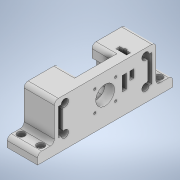
# Autodesk Inventor part: Y_motor_mount
Saved by Autodesk Inventor 2020 (Build 240168000, 168)
## iProperties
Created: 2022-04-26
Part Number: Y_motor_mount
Material: Ogólny
Document SubType Name: Modeling
Designer: mikoma
Density: 1 g/cm^3
Appearance: Domyślna
Author: mikoma
Autodesk Inventor part; units mm, degrees
ref_plane "YZ Plane" through (0, 0, 0) normal (1, 0, 0) x (0, 1, 0)
ref_plane "XZ Plane" through (0, 0, 0) normal (0, 1, 0) x (-1, 0, 0)
ref_plane "XY Plane" through (0, 0, 0) normal (0, 0, 1) x (1, 0, 0)
sketch "Szkic1" plane through (0, 0, 0) normal (1, 0, 0) x (0, 1, 0)
  circle A0 centre (0, 0) radius 14
  arc A1 (15.7574, 63.5) -> (15.0197, 62.3339) centre (20, 60) ccw construction
  arc A2 (-20.25, 65.4943) -> (-15.0197, 62.3339) centre (-20, 60) ccw
  line L0 (20.25, 69.5) -> (-20.25, 69.5)
  line L1 (-20.25, 69.5) -> (-20.25, 65.4943)
  line L2 (-20.25, 63.5) -> (-15.7574, 63.5) construction
  line L3 (20.25, 63.5) -> (20.25, 65.4943) construction
  line L4 (15.7574, 63.5) -> (20.25, 63.5) construction
  line L5 (20.25, 65.4943) -> (20.25, 69.5)
  line L6 (-20.25, 65.4943) -> (-20.25, 63.5) construction
  line L7 (-15.7574, 63.5) -> (-13, 63.5) construction
  arc A3 (20.25, 65.4943) -> (15.7574, 63.5) centre (20, 60) ccw construction
  arc A4 (-15.7574, 63.5) -> (-20.25, 65.4943) centre (-20, 60) ccw construction
  line L8 (-15.0197, 62.3339) -> (-13, 63.5)
  line L9 (13, 63.5) -> (15.0197, 62.3339)
  arc A5 (15.0197, 62.3339) -> (20.25, 65.4943) centre (20, 60) ccw
  line L10 (13, 63.5) -> (15.7574, 63.5) construction
  arc A6 (-15.0197, 62.3339) -> (-15.7574, 63.5) centre (-20, 60) ccw construction
  line L11 (-13, 63.5) -> (13, 63.5)
  line L12 (14, 0) -> (-14, 0) construction
  arc A7 (15.0197, -62.3339) -> (15.7574, -63.5) centre (20, -60) ccw construction
  arc A8 (-15.0197, -62.3339) -> (-20.25, -65.4943) centre (-20, -60) ccw
  line L13 (20.25, -69.5) -> (-20.25, -69.5)
  line L14 (-20.25, -69.5) -> (-20.25, -65.4943)
  line L15 (-20.25, -63.5) -> (-15.7574, -63.5) construction
  line L16 (20.25, -63.5) -> (20.25, -65.4943) construction
  line L17 (15.7574, -63.5) -> (20.25, -63.5) construction
  line L18 (20.25, -65.4943) -> (20.25, -69.5)
  line L19 (-20.25, -65.4943) -> (-20.25, -63.5) construction
  line L20 (-15.7574, -63.5) -> (-13, -63.5) construction
  arc A9 (15.7574, -63.5) -> (20.25, -65.4943) centre (20, -60) ccw construction
  arc A10 (-20.25, -65.4943) -> (-15.7574, -63.5) centre (-20, -60) ccw construction
  line L21 (-15.0197, -62.3339) -> (-13, -63.5)
  line L22 (13, -63.5) -> (15.0197, -62.3339)
  arc A11 (20.25, -65.4943) -> (15.0197, -62.3339) centre (20, -60) ccw
  line L23 (13, -63.5) -> (15.7574, -63.5) construction
  arc A12 (-15.7574, -63.5) -> (-15.0197, -62.3339) centre (-20, -60) ccw construction
  line L24 (-13, -63.5) -> (13, -63.5)
  line L25 (24.5, 75.5) -> (-19, 75.5)
  line L26 (-40, 75.5) -> (-40, -75.5)
  line L27 (-19, -75.5) -> (24.5, -75.5)
  line L28 (30.5, -69.5) -> (30.5, -31.5)
  arc A13 (30.5, 69.5) -> (24.5, 75.5) centre (24.5, 69.5) ccw
  arc A14 (24.5, -75.5) -> (30.5, -69.5) centre (24.5, -69.5) ccw
  line L29 (-40, 75.5) -> (-25, 75.5) construction
  line L30 (-25, 81.5) -> (-25, 94.5)
  line L31 (-31, 100.5) -> (-40, 100.5)
  line L32 (-40, 100.5) -> (-40, 75.5)
  arc A15 (-25, 94.5) -> (-31, 100.5) centre (-31, 94.5) ccw
  arc A16 (-25, 81.5) -> (-19, 75.5) centre (-19, 81.5) ccw
  line L33 (-40, -75.5) -> (-25, -75.5) construction
  line L34 (-25, -81.5) -> (-25, -94.5)
  line L35 (-31, -100.5) -> (-40, -100.5)
  line L36 (-40, -100.5) -> (-40, -75.5)
  arc A17 (-31, -100.5) -> (-25, -94.5) centre (-31, -94.5) ccw
  arc A18 (-19, -75.5) -> (-25, -81.5) centre (-19, -81.5) ccw
  circle A19 centre (15.5, 15.5) radius 1.75
  circle A20 centre (15.5, -15.5) radius 1.75
  circle A21 centre (-15.5, 15.5) radius 1.75
  circle A22 centre (-15.5, -15.5) radius 1.75
  line L37 (15.5, -15.5) -> (-15.5, 15.5) construction
  line L38 (15.5, 15.5) -> (-15.5, -15.5) construction
  circle A23 centre (15.5, 15.5) radius 3.5
  circle A24 centre (15.5, -15.5) radius 3.5
  circle A25 centre (-15.5, -15.5) radius 3.5
  circle A26 centre (-15.5, 15.5) radius 3.5
  line L39 (24.5, -25.5) -> (-15.5, -25.5)
  line L40 (-21.5, -19.5) -> (-21.5, 19.5)
  line L41 (-15.5, 25.5) -> (24.5, 25.5)
  line L42 (30.5, 25.5) -> (30.5, -25.5) construction
  arc A27 (30.5, -31.5) -> (24.5, -25.5) centre (24.5, -31.5) ccw
  arc A28 (-21.5, -19.5) -> (-15.5, -25.5) centre (-15.5, -19.5) ccw
  arc A29 (-15.5, 25.5) -> (-21.5, 19.5) centre (-15.5, 19.5) ccw
  line L43 (30.5, 31.5) -> (30.5, 69.5)
  arc A30 (24.5, 25.5) -> (30.5, 31.5) centre (24.5, 31.5) ccw
  line L44 (30.5, -31.5) -> (30.5, 31.5)
  point P0 (-25, 100.5)
  point P1 (-25, -100.5)
  dimension "d0" = 28
  dimension "d1" = 11
  dimension "d2" = 40
  dimension "d3" = 20
  dimension "d4" = 60
  dimension "d6" = 6
  dimension "d8" = 3.5
  dimension "d9" = 150
  dimension "d10" = 150
  dimension "d11" = 26
  dimension "d12" = 13
  dimension "d13" = 6
  dimension "d14" = 6
  dimension "d15" = 10.5
  dimension "d16" = 20
  dimension "d17" = 6
  dimension "d18" = 15
  dimension "d19" = 25
  dimension "d20" = 6
  dimension "d21" = 15
  dimension "d22" = 25
  dimension "d23" = 6
  dimension "d24" = 3.5
  dimension "d25" = 31
  dimension "d26" = 31
  dimension "d27" = 7
  dimension "d34" = 10
  dimension "d35" = 10
  dimension "d36" = 6
  dimension "d37" = 6
  dimension "d38" = 6
  dimension "d50" = 0.25
  dimension "d51" = 0.25
  constraints: 90 end point, 46 point on circle, 31 centre point, 20 tangent, 17 parallel, 14 symmetric about line, 13 point on line, 12 equal radius, 6 horizontal, 6 perpendicular, 5 coincident, 4 horizontal alignment, 2 midpoint, 2 vertical alignment, 1 collinear, 1 vertical, 6 other
  measures "d0" diameter of A0
  measures "d1" diameter of A1
  measures "d2" distance of A2.centre A1.centre
  measures "d3" horizontal distance of point (0, 0) A1.centre
  measures "d4" vertical distance of A1.centre point (0, 0)
  measures "d6" distance of L3.start L0.start
  measures "d8" distance from line of L2 A1.centre
  measures "d9" angle of L8 L7
  measures "d10" angle of L7 L9
  measures "d11" distance of L7.end L9.start
  measures "d12" horizontal distance of L9.start point (0, 0)
  measures "d13" distance between parallel lines of L0 L25
  measures "d14" distance between parallel lines of L13 L27
  measures "d15" distance from line of A1.centre L28
  measures "d16" distance from line of A2.centre L26
  measures "d17" radius of A13
  measures "d18" distance of point (-25, 100.5) L31.end
  measures "d19" distance of L29.end point (-25, 100.5)
  measures "d20" radius of A15
  measures "d21" distance of point (-25, -100.5) L35.end
  measures "d22" distance of L33.end point (-25, -100.5)
  measures "d23" radius of A17
  measures "d24" diameter of A19
  measures "d25" distance of L37.start L38.start
  measures "d26" distance of L38.end L37.start
  measures "d27" diameter of A23
  measures "d34" distance from line of L39 A24.centre
  measures "d35" distance from line of A23.centre L41
  measures "d36" distance from line of L38.end L40
  measures "d37" radius of A27
  measures "d38" radius of A30
  measures "d50" distance from line of A1.centre L5
  measures "d51" distance from line of L1 A2.centre
extrude "Wyciągnięcie proste1" add sketch "Szkic1" along normal blind 45 contours A0 | L1 L0 L5 A5 L9 L11 L8 A2 | L21 L24 L22 A11 L18 L13 L14 A8 | A13 L43 A30 L41 A29 L40 A28 L39 A27 L28 A14 L27 A18 L34 A17 L35 L36 L26 L32 L31 A15 L30 A16 L25 | L44 A27 L39 A28 L40 A29 L41 A30 | A19 | A20 | A21 | A22 | A23 | A24 | A25 | A26
extrude "Wyciągnięcie proste2" cut sketch "Szkic1" along normal blind 31 contours A0 | L44 A27 L39 A28 L40 A29 L41 A30 | A19 | A20 | A21 | A22 | A23 | A24 | A25 | A26
extrude "Wyciągnięcie proste12" cut sketch "Szkic1" along normal through all contours L1 L0 L5 A5 L9 L11 L8 A2 | L21 L24 L22 A11 L18 L13 L14 A8
extrude "Wyciągnięcie proste4" cut sketch "Szkic1" along normal through all contours A0 | A19 | A20 | A21 | A22
sketch "Szkic2" plane through (0, -25, 94.5) normal (0, 1, 0) x (1, 0, 0)
  circle A0 centre (37, 6.5) radius 5.5
  circle A1 centre (8, 6.5) radius 5.5
  circle A2 centre (37, 6.5) radius 3.25
  circle A3 centre (8, 6.5) radius 3.25
  line L0 (45, 13) -> (45, 0) projected
  line L1 (0, -6) -> (45, -6) projected
  line L2 (0, 13) -> (0, 0) projected
  point P0 (0, 94.5)
  dimension "d41" = 6.5
  dimension "d42" = 11
  dimension "d43" = 8
  dimension "d44" = 12.5
  dimension "d45" = 8
  constraints: 4 centre point, 2 coincident, 2 equal radius, 1 horizontal alignment
  measures "d41" diameter of A2
  measures "d42" diameter of A0
  measures "d43" distance from line of A0.centre L0
  measures "d44" distance from line of L1 A0.centre
  measures "d45" distance from line of L2 A1.centre
extrude "Wyciągnięcie proste5" cut sketch "Szkic2" against normal through all contours A2 | A3
extrude "Wyciągnięcie proste6" cut sketch "Szkic2" against normal blind 5
mirror "Odbij1" about plane through (0, 0, 0) normal (0, 0, 1) of "Wyciągnięcie proste6", "Wyciągnięcie proste5"
sketch "Szkic5" plane through (0, -15.5, -25.5) normal (0, 0, 1) x (1, 0, 0)
  circle A0 centre (8, 22.5) radius 1.75
  circle A1 centre (8, 12.5) radius 1.75
  line L0 (0, 0) -> (0, 40) projected
  line L1 (31, 46) -> (0, 46) projected
  line L2 (31, 46) -> (0, 46) projected
  line L3 (0, 46) -> (45, 46) projected
  line L4 (0, 46) -> (45, 46) projected
  point P0 (0, 15.5)
  dimension "d63" = 3.5
  dimension "d64" = 3.5
  dimension "d65" = 8
  dimension "d66" = 10
  dimension "d67" = 23.5
  constraints: 2 centre point, 1 vertical alignment
  measures "d63" diameter of A0
  measures "d64" diameter of A1
  measures "d65" distance from line of L0 A0.centre
  measures "d66" distance of A1.centre A0.centre
  measures "d67" distance from line of A0.centre L1
extrude "Wyciągnięcie proste8" cut sketch "Szkic5" against normal blind 20
sketch "Szkic3" plane through (0, 0, 0) normal (-1, 0, 0) x (0, 0, 1)
  line L0 (-25.5, -15.5) -> (-25.5, 24.5) projected
  line L1 (-25.5, 12.5) -> (-32, 12.5)
  line L2 (-32, 12.5) -> (-32, -8.5)
  line L3 (-32, -8.5) -> (-25.5, -8.5)
  line L4 (-25.5, -8.5) -> (-25.5, 12.5)
  line L5 (-69.5, 30.5) -> (-31.5, 30.5) projected
  line L6 (-41, 10) -> (-38.4, 10)
  line L7 (-38.4, 10) -> (-38.4, 4)
  line L8 (-38.4, 4) -> (-41, 4)
  line L9 (-41, 4) -> (-41, 10)
  line L10 (-41, 0) -> (-38.4, 0)
  line L11 (-38.4, 0) -> (-38.4, -6)
  line L12 (-38.4, -6) -> (-41, -6)
  line L13 (-41, -6) -> (-41, 0)
  point P0 (0, 0)
  dimension "d52" = 21
  dimension "d53" = 6.5
  dimension "d54" = 18
  dimension "d55" = 2.6
  dimension "d56" = 6
  dimension "d57" = 6
  dimension "d58" = 2.5
  dimension "d59" = 2.5
  dimension "d60" = 9
  constraints: 24 end point, 6 parallel, 3 horizontal, 3 perpendicular, 2 vertical alignment, 1 point on line
  measures "d52" distance of L1.end L2.end
  measures "d53" distance of L1.start L1.end
  measures "d54" distance between parallel lines of L1 L5
  measures "d55" distance of L6.start L6.end
  measures "d56" distance of L8.end L6.start
  measures "d57" distance of L12.end L10.start
  measures "d58" distance between parallel lines of L1 L6
  measures "d59" distance between parallel lines of L3 L12
  measures "d60" distance between parallel lines of L2 L9
extrude "Wyciągnięcie proste7" cut sketch "Szkic3" against normal through all contours L3 L2 L1 L0
extrude "Wyciągnięcie proste9" cut sketch "Szkic3" against normal blind 11 contours L6 L7 L8 L9 | L10 L11 L12 L13
sketch "Szkic6" plane through (0, 30.5, 69.5) normal (0, 1, 0) x (1, 0, 0)
  line L0 (24, 106.5) -> (40, 106.5)
  line L1 (40, 106.5) -> (40, 112.3)
  line L2 (40, 112.3) -> (34, 112.3)
  line L3 (24, 112.3) -> (24, 106.5)
  line L4 (34, 112.3) -> (34, 114)
  line L5 (34, 114) -> (30, 114)
  line L6 (30, 114) -> (30, 112.3)
  line L7 (0, 101.5) -> (45, 101.5) projected
  line L8 (0, 101.5) -> (45, 101.5) projected
  line L9 (6.25, 101.5) -> (9.75, 101.5) projected
  line L10 (6.25, 101.5) -> (9.75, 101.5) projected
  line L11 (45, 139) -> (45, 0) projected
  line L12 (30, 112.3) -> (24, 112.3)
  line L13 (34, 112.3) -> (30, 112.3) construction
  point P0 (0, 69.5)
  dimension "d77" = 5.8
  dimension "d79" = 4
  dimension "d80" = 1.7
  dimension "d81" = 6
  dimension "d82" = 16
  dimension "d83" = 5
  dimension "d84" = 5
  constraints: 18 end point, 6 parallel, 1 horizontal, 1 perpendicular
  measures "d77" distance of L0.end L1.end
  measures "d79" distance of L4.end L5.end
  measures "d80" distance of L2.end L4.end
  measures "d81" distance between parallel lines of L1 L4
  measures "d82" distance of L0.start L0.end
  measures "d83" distance from line of L0.start L8
  measures "d84" distance between parallel lines of L11 L1
extrude "Wyciągnięcie proste10" cut sketch "Szkic6" against normal blind 30
sketch "Szkic7" plane through (45, 0, 0) normal (1, 0, 0) x (0, 0, -1)
  line L0 (42.8, 30.5) -> (37, 30.5) projected
  line L1 (42.8, 30.5) -> (42.8, 0.5) projected
  line L2 (42.8, 0.5) -> (37, 0.5) projected
  line L3 (37, 30.5) -> (37, 0.5) projected
  line L4 (42.8, 0.5) -> (37, 0.5) projected
  line L5 (42.8, 30.5) -> (42.8, 0.5) projected
  line L6 (37, 0.5) -> (42.8, 0.5)
  line L7 (42.8, 0.5) -> (42.8, 12.5)
  line L8 (42.8, 12.5) -> (37, 12.5)
  line L9 (37, 12.5) -> (37, 0.5)
  point P0 (0, 0)
  point P1 (37, 12.5)
  dimension "d87" = 12
  constraints: 8 end point, 2 parallel, 1 horizontal, 1 perpendicular, 1 point on line
  measures "d87" distance between parallel lines of L2 L8
extrude "Wyciągnięcie proste11" cut sketch "Szkic7" against normal up to next contours L1 L2 L3 L8
equation "\"d3\" = 0.5 * d2"
equation "\"d12\" = 0.5 * d11"
equation "\"d14\" = d13"
equation "\"d38\" = d37"
